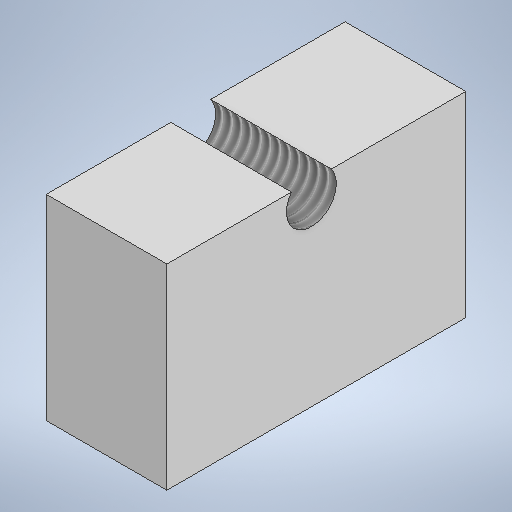
# Autodesk Inventor part: Proyecto 1
Saved by Autodesk Inventor 2025.1 (Build 291241000, 241)
## iProperties
Created: 2024-10-04
Part Number: Proyecto 1
Material: Genérico
Document SubType Name: Sheet Metal
Designer: Octavio
Density: 1 g/cm^3
Sheet Metal Rule: Por defecto_mm
Appearance: Valor por defecto
Author: Octavio
Autodesk Inventor part; units mm, degrees
ref_plane "YZ Plane" through (0, 0, 0) normal (1, 0, 0) x (0, 1, 0)
ref_plane "XZ Plane" through (0, 0, 0) normal (0, 1, 0) x (-1, 0, 0)
ref_plane "XY Plane" through (0, 0, 0) normal (0, 0, 1) x (1, 0, 0)
sketch "Boceto1" plane through (0, 0, 0) normal (1, 0, 0) x (0, 1, 0)
  line L0 (7.6041, 11.4062) -> (-8.6387, 11.4062)
  line L1 (-8.6387, 11.4062) -> (-8.6387, -13.3718)
  line L2 (-8.6387, -13.3718) -> (7.6041, -13.3718)
  line L3 (7.6041, -13.3718) -> (7.6041, 11.4062)
  point P0 (0, 0)
  constraints: 8 end point, 2 parallel, 1 horizontal, 1 perpendicular
extrude "Extrusión1" add sketch "Boceto1" along normal blind 10
sketch "Boceto2" plane through (10, 0, 0) normal (1, 0, 0) x (0, 0, -1)
  line L0 (13.3718, -8.6387) -> (13.3718, 7.6041) projected
  line L1 (-11.4062, -8.6387) -> (13.3718, -8.6387) projected
  point P0 (0, 0)
  point P1 (0.575, 6.3613)
  point P2 (13.3718, -0.5173)
  dimension "d9" = 12.7969
  dimension "d10" = 15
  constraints: 1 midpoint
  measures "d9" horizontal distance of point (13.372, -0.517) point (0.575, 6.361)
  measures "d10" distance from line of L1 point (0.575, 6.361)
hole "Agujero1" at (10, 6.3613, -0.575) direction (-1, 0, 0) diameter 4.134 end through all thread size "M5x0.8" class "6H" standard "ISO Metric profile"
equation "\"Radio_pliegue\" = Grosor"
equation "\"Anchura_desahogo_plegado\" = Grosor"
equation "\"Profundidad_desahogo_plegado\" = 0.5 * Grosor"
equation "\"Tamaño_destalonado\" = 4 * Grosor"
equation "\"Remanente_mínimo\" = 2 * Grosor"
equation "\"Radiodetransición\" = Radio_pliegue"
equation "\"Tamaño_de_radio_de_Jacobi\" = Radio_pliegue"
equation "\"TamañoSeparación\" = Grosor"
equation "\"Grosor\" = 0.5"
